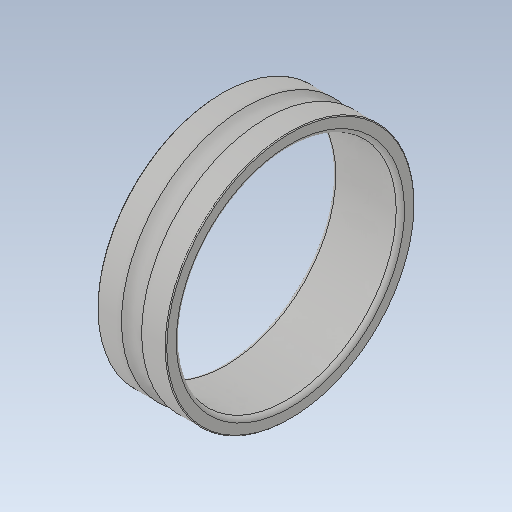
# Autodesk Inventor part: SKF_W 617/8_PART1
Saved by Autodesk Inventor 2021.4 (Build 254397000, 397)
## iProperties
Created: 2022-07-06
Part Number: SKF_W 617/8_PART1
Material: Generic
Catalog Web Link: www.cadenas.de
Description: -Deep groove ball bearings
Vendor: SKF
Document SubType Name: Modeling
Designer: psAdmin
Manufacturer: SKF
Mass: 1 g
Surface Area: 1.59253 cm^2
Volume: 0.0331388 cm^3
Density: 1 g/cm^3
Appearance: PSOLRGB-175-175-175
Category: PARTsolutions
Company: SKF
PSOL_IDENT_0: {$CADENAS_DATA/23d-libs/skf/bearings_units_and_housings/ball_bearings/deep_groove_ball_bearings/bb1_
PSOL_IDENT_1: 001_101.prj},201 {VTYP=3D},{NB=SKF_W 617/8_PART1},{LINA=SKF_W 617/8_PART1},{NN=BB1_001_101_PART1},{N
PSOL_IDENT_2: OPRJ=TRUE},{DATE=10.06.2022 10:28:37},{GEOMDATE=31.05.2022 11:14:58},{VERSION=},{LINEID=17920},{WBVA
PSOL_IDENT_3: R=},{WBNUMERIC=}  {NB=SKF_W 617/8_PART1},{LINA=SKF_W 617/8_PART1},{KT=DUMMY},{DESIGNATION=W 617/8},{
PSOL_IDENT_4: R12=0.15},{DD=8.000},{D=12.000},{B=2.500},{C=},{CX=},{CXX=},{CA=0.000},{XXVARIANT=},{XXDESIGN=Single
PSOL_IDENT_5: row stainless steel},{XXSEALING=No seals},{DESIGN=dgbbw},{DESIGNIR=dgbbw},{VARIANT=},{DD1=9.05},{DD
PSOL_IDENT_6: 2=},{DD2X=},{DD2A=0.00},{D1=10.90},{D1X=0.00},{D2=},{D2A=0.00},{D3=},{D3X=},{D3A=0.000},{D4=},{HH=0.
PSOL_IDENT_7: 000},{BB=0.000},{BBX=},{BBA=0.000},{FF=},{R0MAX=0.000},{R0=0.000},{PITCH=10.00},{DW=1.200},{DDAMIN=9
PSOL_IDENT_8: .000},{DDAMAX=0.000},{DDBMIN=0.000},{DDBMAX=0.000},{DBMIN=0.000},{DAMAX=11.000},{BBAMIN=0.000},{CAMA
PSOL_IDENT_9: X=0.000},{RAMAX=0.150},{LOAD1=0.312},{LOAD2=0.140},{LOAD3=0.006},{SPEED1=100000},{SPEED2=63000},{KR=
PSOL_IDENT_10: 0.015},{F0=8.200},{Z=12},{II=1},{MASS=0.001},{BEARING=W 617/8},{RING=},{HELP=0.550},{HELP2=0.550},{D
PSOL_IDENT_11: D1ALG=4.525},{YALG=4.525},{PITCH1=10.000},{DW1=1.200},{YALG1=5.450},{HALG1=0.550},{SH=4.525},{CU=0.2
PSOL_IDENT_12: 60},{HALG=0.525},{B1=0},{SHIELDHELP=1},{D4A=0.000},{FFA=0.000},{RS1=},{HELP3=0}
NB: SKF_W 617/8_PART1
NT: Deep groove ball bearings
NBSYN: SKF_$DESIGNATION._PART1
LINA: SKF_W 617/8_PART1
CATALOG: SKF
DESIGNATION: W 617/8
R12: 0.15
DD: 8
D: 12
B: 2.5
XXDESIGN: Single row stainless steel
XXSEALING: No seals
LOAD1: 0.312
LOAD2: 0.14
LOAD3: 0.006
SPEED1: 100000
SPEED2: 63000
BEARING: W 617/8
SUPPLIER: SKF
ARTICLENO: SKF_W 617/8_PART1
BOMINFO: SKF_W 617/8_PART1
CREATOR: CADENAS GmbH
Title: SKF_W 617/8_PART1
Author: Cadenas PARTsolutions
Comments: Deep groove ball bearings
Autodesk Inventor part; units mm, degrees
ref_plane "YZ Plane" through (0, 0, 0) normal (1, 0, 0) x (0, 1, 0)
ref_plane "XZ Plane" through (0, 0, 0) normal (0, 1, 0) x (-1, 0, 0)
ref_plane "XY Plane" through (0, 0, 0) normal (0, 0, 1) x (1, 0, 0)
sketch "Sketch_10" plane through (0, 0, 0) normal (0, 0, 1) x (1, 0, 0)
  line L0 (50, 0) -> (-50, 0)
  line L1 (0, 4.495) -> (0, 4.15)
  arc A0 (0, 4.15) -> (0.15, 4) centre (0.15, 4.15) ccw
  line L2 (0.15, 4) -> (2.35, 4)
  arc A1 (2.35, 4) -> (2.5, 4.15) centre (2.35, 4.15) ccw
  line L3 (2.5, 4.15) -> (2.5, 4.495)
  arc A2 (2.5, 4.495) -> (2.47, 4.525) centre (2.47, 4.495) ccw
  line L4 (2.47, 4.525) -> (1.6166, 4.525)
  arc A3 (0.8834, 4.525) -> (1.6166, 4.525) centre (1.25, 5) ccw
  line L5 (0.8834, 4.525) -> (0.03, 4.525)
  arc A4 (0.03, 4.525) -> (0, 4.495) centre (0.03, 4.495) ccw
  constraints: 12 end point, 10 point on circle, 5 centre point
revolve "Revolution1" add sketch "Sketch_10" angle 360 about axis through (50, 0, 0) along (1, 0, 0)
body "Solid1"
